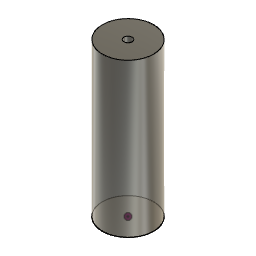
Veroboard Drill Handler (Autodesk Fusion 360 design; units mm, degrees)
Autodesk Fusion 360 part; units mm, degrees
sketch "Sketch1" plane through (0, 0, 0) normal (0, 0, 1) x (1, 0, 0)
  circle A0 centre (0, 0) radius 7.5
  dimension "d13" = 15
  constraint coincident A0.centre origin
  measures "d13" diameter of A0
extrude "Extrude4" add sketch "Sketch1" along normal blind 45
sketch "Sketch3" plane through (0, 0, 45) normal (0, 0, 1) x (-1, 0, 0)
  circle A0 centre (0, 0) radius 7.5
  circle A1 centre (0, 0) radius 1.2
  dimension "d16" = 2.4
  constraint coincident A0.centre A1.centre
  measures "d16" diameter of A1
extrude "Extrude5" cut sketch "Sketch3" against normal blind 35 contours A1
equation "drill_hole_radius = 1.2 mm"
equation "handle_length = 45 mm"
equation "handle_radius = 7.5 mm"
equation "drill_hole_length = 35 mm"
equation "d13 = handle_radius * 2"
equation "d14 = handle_length"
equation "d16 = drill_hole_radius * 2"
equation "d17 = -drill_hole_length"
